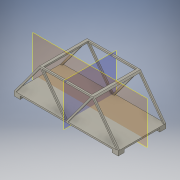
# Autodesk Inventor part: bridge
Saved by Autodesk Inventor 2019 (Build 230136000, 136)
## iProperties
Created: 2020-01-16
Part Number: bridge
Material: Generic
Document SubType Name: Modeling
Designer: tguillod
Density: 1 g/cm^3
Appearance: Steel - Cast
Author: tguillod
Autodesk Inventor part; units mm, degrees
ref_plane "YZ Plane" through (0, 0, 0) normal (1, 0, 0) x (0, 1, 0)
ref_plane "XZ Plane" through (0, 0, 0) normal (0, 1, 0) x (-1, 0, 0)
ref_plane "XY Plane" through (0, 0, 0) normal (0, 0, 1) x (1, 0, 0)
sketch "Sketch1" plane through (0, 0, 0) normal (0, 0, 1) x (1, 0, 0)
  line L0 (0, 0) -> (7000, 0)
  line L1 (7000, 0) -> (7000, 100)
  line L2 (0, 100) -> (0, 0)
  line L3 (1700, 2400) -> (5300, 2400)
  line L4 (0, 100) -> (1700, 2400)
  line L5 (1750.4378, 2300) -> (124.3509, 100)
  line L6 (5300, 2400) -> (7000, 100)
  line L7 (6875.6491, 100) -> (5249.5622, 2300)
  line L8 (3500, 100) -> (1874.7657, 2300)
  line L9 (3500, 100) -> (5125.2343, 2300)
  line L10 (1750.4378, 2300) -> (3375.6722, 100)
  line L11 (5125.2343, 2300) -> (1874.7657, 2300)
  line L12 (5249.5622, 2300) -> (3624.3278, 100)
  line L13 (6875.6491, 100) -> (3624.3278, 100)
  line L14 (3375.6722, 100) -> (124.3509, 100)
  dimension "d15" = 100
  dimension "d16" = 100
  dimension "d17" = 100
  dimension "d18" = 100
  dimension "d19" = 100
  dimension "d20" = 100
  dimension "d21" = 100
  dimension "d23" = 1700
  dimension "d25" = 3500
  dimension "d27" = 100
  dimension "d28" = 100
  dimension "d39" = 3500
  dimension "d40" = 2200
  dimension "d42" = 100
  dimension "d50" = 1700
  dimension "d51" = 2300
  dimension "d52" = 2300
  dimension "d53" = 100
  constraints: 30 end point, 8 parallel, 2 horizontal, 1 perpendicular
  measures "d15" distance between parallel lines of L0 L13
  measures "d16" distance between parallel lines of L0 L14
  measures "d17" distance between parallel lines of L6 L7
  measures "d18" distance between parallel lines of L5 L4
  measures "d19" distance between parallel lines of L9 L12
  measures "d20" distance between parallel lines of L8 L10
  measures "d21" distance between parallel lines of L11 L3
  measures "d23" horizontal distance of L2.start L3.start
  measures "d25" distance of L2.start L8.start
  measures "d27" distance from line of L7.end L3
  measures "d28" distance from line of L5.start L3
  measures "d39" horizontal distance of L0.end L8.start
  measures "d40" distance between parallel lines of L14 L11
  measures "d42" distance of L0.end L1.end
  measures "d50" horizontal distance of L0.end L3.end
  measures "d51" vertical distance of L2.start L3.start
  measures "d52" vertical distance of L3.end L1.end
  measures "d53" distance from line of L0 L8.start
extrude "Extrusion1" add sketch "Sketch1" along normal blind 100
sketch "Sketch2" plane through (0, 0, 100) normal (0, 0, 1) x (1, 0, 0)
  line L0 (3624.3278, 100) -> (6875.6491, 100) projected
  line L1 (6875.6491, 100) -> (5249.5622, 2300) projected
  line L2 (5249.5622, 2300) -> (3624.3278, 100) projected
  line L3 (3375.6722, 100) -> (1750.4378, 2300) projected
  line L4 (1750.4378, 2300) -> (124.3509, 100) projected
  line L5 (124.3509, 100) -> (3375.6722, 100) projected
  line L6 (1874.7657, 2300) -> (3500, 100) projected
  line L7 (3500, 100) -> (5125.2343, 2300) projected
  line L8 (5125.2343, 2300) -> (1874.7657, 2300) projected
  line L9 (0, 0) -> (0, 100) projected
  line L10 (0, 100) -> (1700, 2400) projected
  line L11 (1700, 2400) -> (5300, 2400) projected
  line L12 (5300, 2400) -> (7000, 100) projected
  line L13 (7000, 100) -> (7000, 0) projected
  line L14 (7000, 0) -> (0, 0) projected
  line L15 (0, 100) -> (7000, 100)
  line L16 (7000, 100) -> (7000, 0)
  line L17 (7000, 0) -> (0, 0)
  line L18 (0, 0) -> (0, 100)
  line L19 (1874.7657, 2300) -> (3500, 100) projected
  line L20 (1874.7657, 2300) -> (1626.087, 2300)
  line L21 (1874.7657, 2300) -> (1874.7657, 2400)
  line L22 (5300, 2400) -> (1700, 2400) projected
  line L23 (1874.7657, 2400) -> (1700, 2400)
  line L24 (1700, 2400) -> (1626.087, 2300)
  line L25 (5125.2343, 2300) -> (3500, 100) projected
  line L26 (5125.2343, 2300) -> (5373.913, 2300)
  line L27 (5373.913, 2300) -> (5300, 2400)
  line L28 (5125.2343, 2300) -> (5125.2343, 2400)
  line L29 (5125.2343, 2400) -> (5300, 2400)
  line L30 (1700, 2400) -> (0, 100) projected
  line L31 (7000, 100) -> (5300, 2400) projected
  constraints: 24 end point, 4 point on line, 3 collinear, 3 parallel, 3 perpendicular, 2 horizontal
extrude "Extrusion6" add sketch "Sketch2" along normal blind 1500 contours L0 L15 L13 L14 L9 L5 | L26 L28 L11 L12 | L20 L10 L11 L21
sketch "Sketch5" plane through (0, 0, 0) normal (0, -1, 0) x (1, 0, 0)
  line L0 (0, 1600) -> (7000, 1600)
  line L1 (7000, 1600) -> (7000, 0) projected
  line L2 (7000, 0) -> (0, 0) projected
  line L3 (0, 0) -> (0, 1600) projected
  line L4 (7000, 1600) -> (0, 1600)
  line L5 (0, 1600) -> (400, 1600)
  line L6 (400, 1600) -> (400, 0)
  line L7 (400, 0) -> (0, 0)
  line L8 (0, 0) -> (0, 1600)
  line L9 (0, 0) -> (7000, 0) projected
  line L10 (7000, 1600) -> (6600, 1600)
  line L11 (6600, 1600) -> (6600, 0)
  line L12 (6600, 0) -> (7000, 0)
  line L13 (7000, 0) -> (7000, 1600)
  dimension "d58" = 400
  dimension "d59" = 400
  constraints: 20 end point, 4 parallel, 2 horizontal, 2 perpendicular, 2 point on line
  measures "d58" distance between parallel lines of L3 L6
  measures "d59" distance between parallel lines of L1 L11
extrude "Extrusion7" add sketch "Sketch5" along normal blind 200 contours L0 L6 L2 L3 | L0 L1 L2 L11
sketch "Sketch6" plane through (0, 0, 1600) normal (0, 0, 1) x (1, 0, 0)
  line L0 (1874.7657, 2400) -> (1874.7657, 2300) projected
  line L1 (1874.7657, 2300) -> (1626.087, 2300) projected
  line L2 (1626.087, 2300) -> (1700, 2400) projected
  line L3 (1700, 2400) -> (1874.7657, 2400) projected
  line L4 (5373.913, 2300) -> (5125.2343, 2300) projected
  line L5 (5125.2343, 2300) -> (5125.2343, 2400) projected
  line L6 (5125.2343, 2400) -> (5300, 2400) projected
  line L7 (5300, 2400) -> (5373.913, 2300) projected
  line L8 (0, 100) -> (7000, 100) projected
  line L9 (7000, 100) -> (7000, -200) projected
  line L10 (7000, -200) -> (6600, -200) projected
  line L11 (6600, -200) -> (6600, 0) projected
  line L12 (6600, 0) -> (400, 0) projected
  line L13 (400, 0) -> (400, -200) projected
  line L14 (400, -200) -> (0, -200) projected
  line L15 (0, -200) -> (0, 100) projected
  line L16 (400, 0) -> (400, -200) projected
  line L17 (400, -200) -> (0, -200) projected
  line L18 (400, 0) -> (0, 0)
  line L19 (0, 0) -> (0, -200)
  line L20 (0, -200) -> (400, -200)
  line L21 (400, -200) -> (400, 0)
  line L22 (400, 0) -> (6600, 0) projected
  line L23 (6600, -200) -> (7000, -200) projected
  line L24 (6600, 0) -> (7000, 0)
  line L25 (7000, 0) -> (7000, -200)
  line L26 (7000, -200) -> (6600, -200)
  line L27 (6600, -200) -> (6600, 0)
  point P0 (0, 0)
  constraints: 16 end point, 4 parallel, 2 horizontal, 2 perpendicular
extrude "Extrusion8" cut sketch "Sketch6" against normal blind 1200 contours L18 L13 L14 L15 | L9 L10 L11 L24
mirror "Mirror4" about plane through (5237.1831, 2344.295, 1600) normal (0, 0, 1)
ref_plane "Work Plane3" through (400, 0, 1600) normal (0, 0, 1) x (1, 0, 0)
ref_plane "Work Plane4" through (3500, 100, 0) normal (-1, 0, 0) x (0, 0, 1)
body "Solid1"
